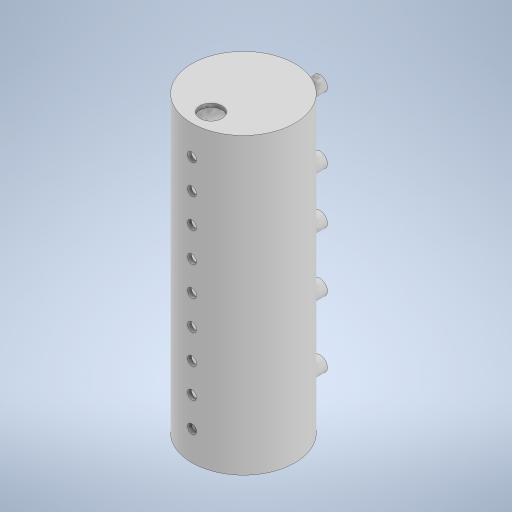
# Autodesk Inventor part: Smoke generator
Saved by Autodesk Inventor 2023 (Build 270158000, 158)
## iProperties
Created: 2022-09-12
Part Number: Smoke generator
Material: Generic
Document SubType Name: Modeling
Designer: earls
Density: 1 g/cm^3
Appearance: Default
Author: earls
Autodesk Inventor part; units mm, degrees
ref_plane "YZ Plane" through (0, 0, 0) normal (1, 0, 0) x (0, 1, 0)
ref_plane "XZ Plane" through (0, 0, 0) normal (0, 1, 0) x (-1, 0, 0)
ref_plane "XY Plane" through (0, 0, 0) normal (0, 0, 1) x (1, 0, 0)
sketch "Sketch1" plane through (0, 0, 0) normal (0, 1, 0) x (-1, 0, 0)
  line L0 (0, 0) -> (0, -19.2268)
  circle A0 centre (0, -19.2268) radius 7.25
  circle A1 centre (0, -35) radius 35
  point P0 (0, -70)
  dimension "d0" = 70
  dimension "d2" = 14.5
  constraints: 2 coincident, 2 end point, 2 vertical alignment, 1 centre point, 1 vertical, 2 other
  measures "d0" distance of point (0, -70) point (0, 0)
  measures "d2" diameter of A0
extrude "Extrusion2" add sketch "Sketch1" along normal mid plane 200 contours A0 | A1
shell "Shell1" thickness 2.5 removed faces 0
sketch "Sketch2" plane through (0, 100, -35) normal (0, 1, 0) x (1, 0, 0)
  circle A0 centre (0, -22.0279) radius 7.5
  point P0 (0, -35)
  dimension "d8" = 15
  constraints: 1 centre point
  measures "d8" diameter of A0
extrude "Extrusion3" cut sketch "Sketch2" against normal blind 2.5
sketch "Sketch3" plane through (0, 0, 0) normal (1, 0, 0) x (0, 1, 0)
  line L0 (-100, -70) -> (100, -70) projected
  line L1 (80, -70) -> (80, -87.1201)
  line L2 (85, -70) -> (85, -87.1201)
  line L3 (100, -70) -> (100, 0) projected
  line L4 (0, -70) -> (0, -87.1201)
  line L5 (-80, -70) -> (-80, -87.1201)
  line L6 (-85, -70) -> (-85, -87.1201)
  line L7 (35, -70) -> (35, -87.1201)
  line L8 (40, -70) -> (40, -87.1201)
  line L9 (-35, -70) -> (-35, -87.1201)
  line L10 (-40, -70) -> (-40, -87.1201)
  line L11 (-100, 0) -> (-100, -70) projected
  line L12 (100, -70) -> (100, 0) projected
  line L13 (85, -87.1201) -> (80, -87.1201)
  line L14 (40, -87.1201) -> (35, -87.1201)
  line L15 (-35, -87.1201) -> (-40, -87.1201)
  line L16 (-80, -87.1201) -> (-85, -87.1201)
  line L17 (-100, -70) -> (100, -70) projected
  line L18 (5, -70) -> (5, -87.1201)
  line L19 (5, -87.1201) -> (0, -87.1201)
  point P0 (0, 0)
  point P1 (40, -78.56)
  dimension "d11" = 5
  dimension "d12" = 15
  dimension "d13" = 5
  dimension "d14" = 40
  dimension "d19" = 5
  constraints: 30 end point, 8 symmetric about line, 6 vertical, 3 point on line, 2 collinear, 2 horizontal, 2 midpoint, 1 perpendicular
  measures "d11" distance between parallel lines of L2 L1
  measures "d12" distance between parallel lines of L2 L3
  measures "d13" distance between parallel lines of L8 L7
  measures "d14" distance from line of point (40, -78.56) L1
  measures "d19" distance between parallel lines of L18 L4
revolve "Revolution1" add sketch "Sketch3" angle 360 about axis through (0, 80, -70) along (0, 0, -1) contours L0 L2 L13 L1
revolve "Revolution2" add sketch "Sketch3" angle 360 about axis through (0, 35, -70) along (0, 0, -1) contours L0 L8 L14 L7
revolve "Revolution3" add sketch "Sketch3" angle 360 about axis through (0, -40, -70) along (0, 0, -1) contours L0 L9 L15 L10
revolve "Revolution4" add sketch "Sketch3" angle 360 about axis through (0, -85, -70) along (0, 0, -1) contours L0 L5 L16 L6
revolve "Revolution5" add sketch "Sketch3" angle 360 about axis through (0, 0, -70) along (0, 0, -1) contours L0 L18 L19 L4
shell "Shell2" thickness 2.5 removed faces 5 at (-0.3214, 79.1807, -87.1201) at (-0.3214, 34.1807, -87.1201) at (-0.3989, -0.8768, -87.1201) at (-0.3214, -40.8193, -87.1201) at (-0.3214, -85.8193, -87.1201)
sketch "Sketch4" plane through (0, 80, -87.1201) normal (0, 0, -1) x (-1, 0, 0)
  circle A0 centre (0, 0) radius 2.5 projected
  circle A1 centre (0, -45) radius 2.5 projected
  circle A2 centre (0, -80) radius 2.5 projected
  circle A3 centre (0, -120) radius 2.5 projected
  circle A4 centre (0, -165) radius 2.5 projected
extrude "Extrusion4" cut sketch "Sketch4" against normal blind 30
sketch "Sketch5" plane through (0, 0, 0) normal (1, 0, 0) x (0, 1, 0)
  line L0 (-100, 0) -> (100, 0) projected
  line L1 (0, 0) -> (0, 5.3077)
  line L2 (3, 0) -> (3, 5.3077)
  line L3 (0, 5.3077) -> (3, 5.3077)
  line L4 (23, 0) -> (23, 5.3077)
  line L5 (20, 0) -> (20, 5.3077)
  line L6 (20, 5.3077) -> (23, 5.3077)
  line L7 (43, 0) -> (43, 5.3077)
  line L8 (40, 0) -> (40, 5.3077)
  line L9 (40, 5.3077) -> (43, 5.3077)
  line L10 (63, 0) -> (63, 5.3077)
  line L11 (60, 0) -> (60, 5.3077)
  line L12 (60, 5.3077) -> (63, 5.3077)
  line L13 (83, 0) -> (83, 5.3077)
  line L14 (80, 0) -> (80, 5.3077)
  line L15 (80, 5.3077) -> (83, 5.3077)
  line L16 (-17, 0) -> (-17, 5.3077)
  line L17 (-20, 0) -> (-20, 5.3077)
  line L18 (-20, 5.3077) -> (-17, 5.3077)
  line L19 (3, 0) -> (3, 5.3077)
  line L20 (0, 0) -> (0, 5.3077)
  line L21 (0, 5.3077) -> (3, 5.3077)
  line L22 (23, 0) -> (23, 5.3077)
  line L23 (20, 0) -> (20, 5.3077)
  line L24 (20, 5.3077) -> (23, 5.3077)
  line L25 (43, 0) -> (43, 5.3077)
  line L26 (40, 0) -> (40, 5.3077)
  line L27 (40, 5.3077) -> (43, 5.3077)
  line L28 (63, 0) -> (63, 5.3077)
  line L29 (60, 0) -> (60, 5.3077)
  line L30 (60, 5.3077) -> (63, 5.3077)
  line L31 (-37, 0) -> (-37, 5.3077)
  line L32 (-40, 0) -> (-40, 5.3077)
  line L33 (-40, 5.3077) -> (-37, 5.3077)
  line L34 (-17, 0) -> (-17, 5.3077)
  line L35 (-20, 0) -> (-20, 5.3077)
  line L36 (-20, 5.3077) -> (-17, 5.3077)
  line L37 (3, 0) -> (3, 5.3077)
  line L38 (0, 0) -> (0, 5.3077)
  line L39 (0, 5.3077) -> (3, 5.3077)
  line L40 (23, 0) -> (23, 5.3077)
  line L41 (20, 0) -> (20, 5.3077)
  line L42 (20, 5.3077) -> (23, 5.3077)
  line L43 (43, 0) -> (43, 5.3077)
  line L44 (40, 0) -> (40, 5.3077)
  line L45 (40, 5.3077) -> (43, 5.3077)
  line L46 (-57, 0) -> (-57, 5.3077)
  line L47 (-60, 0) -> (-60, 5.3077)
  line L48 (-60, 5.3077) -> (-57, 5.3077)
  line L49 (-37, 0) -> (-37, 5.3077)
  line L50 (-40, 0) -> (-40, 5.3077)
  line L51 (-40, 5.3077) -> (-37, 5.3077)
  line L52 (-17, 0) -> (-17, 5.3077)
  line L53 (-20, 0) -> (-20, 5.3077)
  line L54 (-20, 5.3077) -> (-17, 5.3077)
  line L55 (3, 0) -> (3, 5.3077)
  line L56 (0, 0) -> (0, 5.3077)
  line L57 (0, 5.3077) -> (3, 5.3077)
  line L58 (23, 0) -> (23, 5.3077)
  line L59 (20, 0) -> (20, 5.3077)
  line L60 (20, 5.3077) -> (23, 5.3077)
  line L61 (-77, 0) -> (-77, 5.3077)
  line L62 (-80, 0) -> (-80, 5.3077)
  line L63 (-80, 5.3077) -> (-77, 5.3077)
  line L64 (-57, 0) -> (-57, 5.3077)
  line L65 (-60, 0) -> (-60, 5.3077)
  line L66 (-60, 5.3077) -> (-57, 5.3077)
  line L67 (-37, 0) -> (-37, 5.3077)
  line L68 (-40, 0) -> (-40, 5.3077)
  line L69 (-40, 5.3077) -> (-37, 5.3077)
  line L70 (-17, 0) -> (-17, 5.3077)
  line L71 (-20, 0) -> (-20, 5.3077)
  line L72 (-20, 5.3077) -> (-17, 5.3077)
  line L73 (3, 0) -> (3, 5.3077)
  line L74 (0, 0) -> (0, 5.3077)
  line L75 (0, 5.3077) -> (3, 5.3077)
  point P0 (0, 2.6538)
  point P1 (3, 3.2308)
  point P2 (23, 3.2308)
  point P3 (20, 2.6538)
  point P4 (43, 3.2308)
  point P5 (40, 2.6538)
  point P6 (63, 3.2308)
  point P7 (60, 2.6538)
  point P8 (83, 3.2308)
  point P9 (80, 2.6538)
  point P10 (-17, 3.2308)
  point P11 (-20, 2.6538)
  point P12 (3, 3.2308)
  point P13 (0, 2.6538)
  point P14 (23, 3.2308)
  point P15 (20, 2.6538)
  point P16 (43, 3.2308)
  point P17 (40, 2.6538)
  point P18 (63, 3.2308)
  point P19 (60, 2.6538)
  point P20 (-37, 3.2308)
  point P21 (-40, 2.6538)
  point P22 (-17, 3.2308)
  point P23 (-20, 2.6538)
  point P24 (3, 3.2308)
  point P25 (0, 2.6538)
  point P26 (23, 3.2308)
  point P27 (20, 2.6538)
  point P28 (43, 3.2308)
  point P29 (40, 2.6538)
  point P30 (-57, 3.2308)
  point P31 (-60, 2.6538)
  point P32 (-37, 3.2308)
  point P33 (-40, 2.6538)
  point P34 (-17, 3.2308)
  point P35 (-20, 2.6538)
  point P36 (3, 3.2308)
  point P37 (0, 2.6538)
  point P38 (23, 3.2308)
  point P39 (20, 2.6538)
  point P40 (-77, 3.2308)
  point P41 (-80, 2.6538)
  point P42 (-57, 3.2308)
  point P43 (-60, 2.6538)
  point P44 (-37, 3.2308)
  point P45 (-40, 2.6538)
  point P46 (-17, 3.2308)
  point P47 (-20, 2.6538)
  point P48 (3, 3.2308)
  point P49 (0, 2.6538)
  dimension "d28" = 20
  dimension "d31" = 20
  constraints: 150 end point, 26 point on line, 2 horizontal, 2 vertical, 1 midpoint, 1 perpendicular, 216 other
  measures "d28" distance of L2.start L4.start
  measures "d31" distance of L2.start L16.start
revolve "Revolution6" add sketch "Sketch5" angle 360 about axis through (0, 0, 0) along (0, 0, 1) contours L1 L3 L2 L0
revolve "Revolution7" add sketch "Sketch5" angle 360 about axis through (0, 20, 0) along (0, 0, 1) contours L5 L6 L4 L0
revolve "Revolution8" add sketch "Sketch5" angle 360 about axis through (0, 40, 0) along (0, 0, 1) contours L8 L9 L7 L0
revolve "Revolution9" add sketch "Sketch5" angle 360 about axis through (0, 60, 0) along (0, 0, 1) contours L11 L12 L10 L0
revolve "Revolution10" add sketch "Sketch5" angle 360 about axis through (0, 80, 0) along (0, 0, 1) contours L14 L15 L13 L0
revolve "Revolution11" add sketch "Sketch5" angle 360 about axis through (0, -20, 0) along (0, 0, 1) contours L17 L18 L16 L0
revolve "Revolution12" add sketch "Sketch5" angle 360 about axis through (0, -40, 0) along (0, 0, 1) contours L32 L33 L31 L0
revolve "Revolution13" add sketch "Sketch5" angle 360 about axis through (0, -60, 0) along (0, 0, 1) contours L47 L48 L46 L0
revolve "Revolution14" add sketch "Sketch5" angle 360 about axis through (0, -80, 0) along (0, 0, 1) contours L62 L63 L61 L0
sketch "Sketch6" plane through (0, -80, 5.3077) normal (0, 0, 1) x (1, 0, 0)
  circle A0 centre (0, 0) radius 3 projected
  circle A1 centre (0, 20) radius 3 projected
  circle A2 centre (0, 40) radius 3 projected
  circle A3 centre (0, 60) radius 3 projected
  circle A4 centre (0, 80) radius 3 projected
  circle A5 centre (0, 100) radius 3 projected
  circle A6 centre (0, 120) radius 3 projected
  circle A7 centre (0, 140) radius 3 projected
  circle A8 centre (0, 160) radius 3 projected
  constraints: 1 other
extrude "Extrusion5" cut sketch "Sketch6" against normal blind 30
equation "\"d19\" = d13"
body "Solid2"
